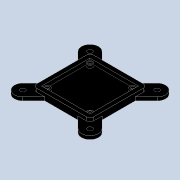
# Autodesk Inventor part: Drok L298 DC Motor Driver Mount
Saved by Autodesk Inventor 2022 (Build 260153000, 153)
## iProperties
Created: 2022-01-02
Part Number: Drok L298 DC Motor Driver Mount
Material: Generic
Document SubType Name: Modeling
Designer: Coy
Density: 1 g/cm^3
Appearance: Anodized - Black
Author: Coy
Autodesk Inventor part; units mm, degrees
ref_plane "YZ Plane" through (0, 0, 0) normal (1, 0, 0) x (0, 1, 0)
ref_plane "XZ Plane" through (0, 0, 0) normal (0, 1, 0) x (-1, 0, 0)
ref_plane "XY Plane" through (0, 0, 0) normal (0, 0, 1) x (1, 0, 0)
sketch "Sketch1" plane through (0, 0, 0) normal (0, 1, 0) x (-1, 0, 0)
  line L0 (0, 0) -> (55.5, 0)
  line L1 (55.5, 0) -> (55.5, 55.5)
  line L2 (55.5, 55.5) -> (0, 55.5)
  line L3 (0, 55.5) -> (0, 0)
  line L4 (-1, 60.5) -> (56.5, 60.5)
  line L5 (60.5, 56.5) -> (60.5, -1)
  line L6 (56.5, -5) -> (-1, -5)
  line L7 (-5, -1) -> (-5, 56.5)
  arc A0 (60.5, 56.5) -> (56.5, 60.5) centre (56.5, 56.5) ccw
  arc A1 (56.5, -5) -> (60.5, -1) centre (56.5, -1) ccw
  arc A2 (-5, -1) -> (-1, -5) centre (-1, -1) ccw
  arc A3 (-1, 60.5) -> (-5, 56.5) centre (-1, 56.5) ccw
  dimension "d0" = 55.5
  dimension "d1" = 55.5
  dimension "d2" = 5
  dimension "d3" = 4
  constraints: 16 end point, 8 point on circle, 8 tangent, 4 centre point, 4 parallel, 3 equal radius, 2 perpendicular, 1 horizontal, 3 other
  measures "d0" distance of L2.end L1.end
  measures "d1" distance of L1.end L0.end
  measures "d2" distance between parallel lines of L2 L4
  measures "d3" radius of A0
extrude "Extrusion1" add sketch "Sketch1" along normal blind 4
sketch "Sketch2" plane through (0, 0, 0) normal (0, -1, 0) x (1, 0, 0)
  line L0 (1, -5) -> (-56.5, -5) projected
  arc A0 (1, -5) -> (5, -1) centre (1, -1) ccw projected
  line L1 (5, 56.5) -> (5, -1) projected
  arc A1 (5, 56.5) -> (1, 60.5) centre (1, 56.5) ccw projected
  line L2 (-56.5, 60.5) -> (1, 60.5) projected
  arc A2 (-56.5, 60.5) -> (-60.5, 56.5) centre (-56.5, 56.5) ccw projected
  line L3 (-60.5, -1) -> (-60.5, 56.5) projected
  arc A3 (-60.5, -1) -> (-56.5, -5) centre (-56.5, -1) ccw projected
  line L4 (0, 0) -> (0, 55.5) projected
  line L5 (-55.5, 0) -> (0, 0) projected
  line L6 (-55.5, 55.5) -> (-55.5, 0) projected
  line L7 (0, 55.5) -> (-55.5, 55.5) projected
  line L8 (-77.75, 77.75) -> (22.25, 77.75) construction
  line L9 (22.25, 77.75) -> (22.25, -22.25) construction
  line L10 (22.25, -22.25) -> (-77.75, -22.25) construction
  line L11 (-77.75, -22.25) -> (-77.75, 77.75) construction
  line L12 (-77.75, 77.75) -> (22.25, -22.25) construction
  line L13 (22.25, 77.75) -> (-77.75, -22.25) construction
  circle A4 centre (10.7227, 66.2227) radius 2.75
  arc A5 (17.617, 59.3284) -> (3.8284, 73.117) centre (10.7227, 66.2227) ccw
  arc A6 (5, 56.5) -> (1, 60.5) centre (1, 56.5) ccw projected
  line L14 (17.617, 59.3284) -> (5, 46.7114)
  line L15 (3.8284, 73.117) -> (-8.7886, 60.5)
  line L16 (-59.3284, 73.117) -> (-46.7114, 60.5)
  arc A7 (-59.3284, 73.117) -> (-73.117, 59.3284) centre (-66.2227, 66.2227) ccw
  circle A8 centre (-66.2227, 66.2227) radius 2.75
  line L17 (-73.117, 59.3284) -> (-60.5, 46.7114)
  line L18 (-73.117, -3.8284) -> (-60.5, 8.7886)
  arc A9 (-73.117, -3.8284) -> (-59.3284, -17.617) centre (-66.2227, -10.7227) ccw
  circle A10 centre (-66.2227, -10.7227) radius 2.75
  line L19 (-59.3284, -17.617) -> (-46.7114, -5)
  line L20 (3.8284, -17.617) -> (-8.7886, -5)
  arc A11 (3.8284, -17.617) -> (17.617, -3.8284) centre (10.7227, -10.7227) ccw
  circle A12 centre (10.7227, -10.7227) radius 2.75
  line L21 (17.617, -3.8284) -> (5, 8.7886)
  point P0 (-27.75, 27.75)
  dimension "d6" = 100
  dimension "d7" = 100
  dimension "d8" = 5.5
  dimension "d9" = 7
  dimension "d12" = 360
  constraints: 28 end point, 8 centre point, 8 point on circle, 4 parallel, 3 point on line, 3 tangent, 2 midpoint, 1 horizontal, 1 perpendicular, 37 other
  measures "d6" distance of L9.end L10.end
  measures "d7" distance of L8.end L9.end
  measures "d8" diameter of A4
  measures "d9" radial gap between concentric circles of A4 A5
extrude "Extrusion2" add sketch "Sketch2" along normal blind 4 contours A0 L1 L21 A11 L20 L0 | L0 A3 L3 A2 L2 A1 L1 A0 | L19 A9 L18 L3 A3 L0 | L1 A1 L2 L15 A5 L14 | L17 A7 L16 L2 A2 L3 | L5 L6 L7 L4
sketch "Sketch3" plane through (0, 0, 0) normal (0, 1, 0) x (1, 0, 0)
  line L0 (-52.25, -52.25) -> (-3.25, -52.25) construction
  line L1 (-3.25, -52.25) -> (-3.25, -3.25) construction
  line L2 (-3.25, -3.25) -> (-52.25, -3.25) construction
  line L3 (-52.25, -3.25) -> (-52.25, -52.25) construction
  line L4 (-52.25, -52.25) -> (-52.25, -55.5) construction
  line L5 (-52.25, -52.25) -> (-55.5, -52.25) construction
  line L6 (-55.5, -55.5) -> (-55.5, 0) construction
  line L7 (-3.25, -3.25) -> (0, -3.25) construction
  line L8 (0, 0) -> (0, -55.5) construction
  line L9 (-3.25, -3.25) -> (-3.25, 0) construction
  line L10 (-55.5, 0) -> (0, 0) construction
  line L11 (0, -55.5) -> (-55.5, -55.5) projected
  circle A0 centre (-52.25, -52.25) radius 3.25
  circle A1 centre (-52.25, -3.25) radius 3.25
  circle A2 centre (-3.25, -3.25) radius 3.25
  circle A3 centre (-3.25, -52.25) radius 3.25
  line L12 (-55.5, 0) -> (0, 0) projected
  line L13 (-55.5, -55.5) -> (-55.5, 0) projected
  line L14 (0, -55.5) -> (-55.5, -55.5) projected
  line L15 (0, 0) -> (0, -55.5) projected
  point P0 (-3.25, 0)
  point P1 (0, -3.25)
  point P2 (0, -52.25)
  point P3 (-3.25, -55.5)
  point P4 (-55.5, -3.25)
  point P5 (-52.25, 0)
  dimension "d16" = 49
  dimension "d17" = 49
  constraints: 16 end point, 5 parallel, 4 coincident, 4 point on line, 2 centre point, 2 horizontal, 2 perpendicular, 1 tangent, 1 vertical, 6 other
  measures "d16" distance of L2.end L1.end
  measures "d17" distance of L1.end L0.end
extrude "Extrusion3" add sketch "Sketch3" along normal blind 2.3 contours L11 A3 L15 | A3 | L11 L13 A0 | A0 | A2 | A2 L12 L15 | L13 L12 A1 | A1
sketch "Sketch4" plane through (0, 2.3, 0) normal (0, 1, 0) x (1, 0, 0)
  arc A0 (0, -52.25) -> (-3.25, -55.5) centre (-3.25, -52.25) ccw projected
  line L0 (0, -3.25) -> (0, -52.25) projected
  arc A1 (-3.25, 0) -> (0, -3.25) centre (-3.25, -3.25) ccw projected
  line L1 (-52.25, 0) -> (-3.25, 0) projected
  arc A2 (-55.5, -3.25) -> (-52.25, 0) centre (-52.25, -3.25) ccw projected
  line L2 (-55.5, -52.25) -> (-55.5, -3.25) projected
  arc A3 (-52.25, -55.5) -> (-55.5, -52.25) centre (-52.25, -52.25) ccw projected
  line L3 (-3.25, -55.5) -> (-52.25, -55.5) projected
  point P0 (0, 0)
extrude "Extrusion4" cut sketch "Sketch4" against normal blind 3
sketch "Sketch5" plane through (0, 2.3, 0) normal (0, 1, 0) x (1, 0, 0)
  line L0 (0, 0) -> (0, -3.25) projected
  line L1 (-3.25, 0) -> (0, 0) projected
  arc A0 (-3.25, 0) -> (0, -3.25) centre (-3.25, -3.25) ccw projected
  arc A1 (0, -52.25) -> (-3.25, -55.5) centre (-3.25, -52.25) ccw projected
  line L2 (0, -55.5) -> (-3.25, -55.5) projected
  line L3 (0, -52.25) -> (0, -55.5) projected
  line L4 (-52.25, -55.5) -> (-55.5, -55.5) projected
  arc A2 (-52.25, -55.5) -> (-55.5, -52.25) centre (-52.25, -52.25) ccw projected
  line L5 (-55.5, -55.5) -> (-55.5, -52.25) projected
  arc A3 (-55.5, -3.25) -> (-52.25, 0) centre (-52.25, -3.25) ccw projected
  line L6 (-55.5, 0) -> (-52.25, 0) projected
  line L7 (-55.5, -3.25) -> (-55.5, 0) projected
  circle A4 centre (-52.25, -52.25) radius 1
  arc A5 (-55.5, -3.25) -> (-52.25, 0) centre (-52.25, -3.25) ccw projected
  circle A6 centre (-52.25, -3.25) radius 1
  arc A7 (-3.25, 0) -> (0, -3.25) centre (-3.25, -3.25) ccw projected
  circle A8 centre (-3.25, -3.25) radius 1
  circle A9 centre (-3.25, -52.25) radius 1
  dimension "d23" = 2
  dimension "d24" = 2
  dimension "d25" = 2
  dimension "d26" = 2
  constraints: 4 centre point, 4 coincident
  measures "d23" diameter of A4
  measures "d24" diameter of A6
  measures "d25" diameter of A8
  measures "d26" diameter of A9
extrude "Extrusion5" cut sketch "Sketch5" against normal up to next contours A4 | A6 | A8 | A9
chamfer "Chamfer1" distance 1 angle 45 4 edges at (-53.25, 2.3, 52.25) (-53.25, 2.3, 3.25) (-4.25, 2.3, 52.25) (-4.25, 2.3, 3.25)
equation "\"d24\" = d23"
equation "\"d25\" = d23"
equation "\"d26\" = d23"
body "Solid1"
